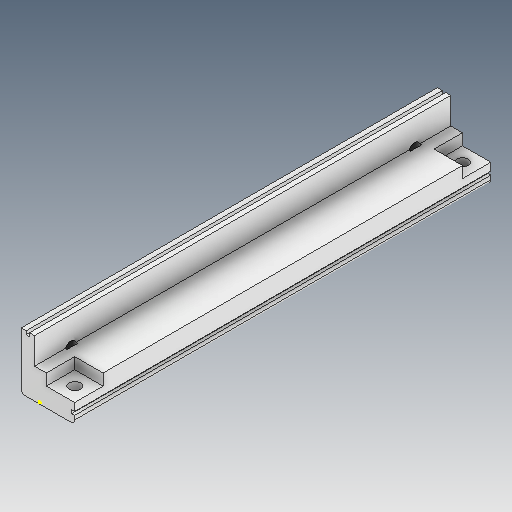
# Autodesk Inventor part: top_edge
Saved by Autodesk Inventor 2027 (Build 310192060, 192F)
## iProperties
Created: 2026-07-26
Part Number: top_edge
Material: ABS Plastic
Document SubType Name: Modeling
Designer: prest
Density: 1.06 g/cm^3
Appearance: Smooth - White
Author: prest
Autodesk Inventor part; units mm, degrees
ref_plane "YZ Plane" through (0, 0, 0) normal (1, 0, 0) x (0, 1, 0)
ref_plane "XZ Plane" through (0, 0, 0) normal (0, 1, 0) x (-1, 0, 0)
ref_plane "XY Plane" through (0, 0, 0) normal (0, 0, 1) x (1, 0, 0)
sketch "Sketch1" plane through (0, 0, 0) normal (0, 1, 0) x (-1, 0, 0)
  line L0 (18.1065, 110) -> (-18.1065, 110)
  line L1 (-18.1065, 110) -> (-18.1065, -110)
  line L2 (-18.1065, -110) -> (18.1065, -110)
  line L3 (18.1065, -110) -> (18.1065, 110)
  point P0 (0, 0)
  point P1 (0, 110)
  point P2 (18.1065, 0)
  dimension "d0" = 220
  dimension "d1" = 36.213
  constraints: 8 end point, 2 midpoint, 2 parallel, 1 horizontal, 1 horizontal alignment, 1 perpendicular, 1 vertical alignment
  measures "d0" distance of L2.end L0.start
  measures "d1" distance of L0.start L0.end
extrude "Extrusion1" add sketch "Sketch1" along normal blind 15
sketch "Sketch2" plane through (0, 15, 0) normal (0, 1, 0) x (1, 0, 0)
  line L0 (-18.1065, 110) -> (-18.1065, -110) projected
  line L1 (18.1065, 110) -> (-18.1065, 110) projected
  line L2 (-18.1065, -110) -> (-3.1065, -110)
  line L3 (-3.1065, -110) -> (-3.1065, 110)
  line L4 (-3.1065, 110) -> (-18.1065, 110)
  line L5 (-18.1065, 110) -> (-18.1065, -110)
  point P0 (0, 0)
  dimension "d4" = 15
  constraints: 8 end point, 2 parallel, 1 horizontal, 1 perpendicular, 1 point on line
  measures "d4" distance of L4.end L3.end
extrude "Extrusion2" add sketch "Sketch2" along normal blind 14
sketch "Sketch3" plane through (0, 15, 0) normal (0, 1, 0) x (1, 0, 0)
  line L0 (-18.1065, -110) -> (18.1065, -110) projected
  line L1 (18.1065, -110) -> (3.1065, -110)
  line L2 (3.1065, -110) -> (3.1065, -95)
  line L3 (3.1065, -95) -> (18.1065, -95)
  line L4 (18.1065, -95) -> (18.1065, -110)
  point P0 (0, 0)
  dimension "d7" = 15
  dimension "d8" = 15
  constraints: 8 end point, 2 parallel, 1 horizontal, 1 perpendicular
  measures "d7" distance of L2.end L3.end
  measures "d8" distance of L1.end L2.end
extrude "Extrusion3" cut sketch "Sketch3" against normal blind 6
mirror "Mirror1" about plane through (0, 0, 0) normal (0, 0, 1) of "Extrusion3"
sketch "Sketch4" plane through (0, 9, 0) normal (0, 1, 0) x (1, 0, 0)
  line L0 (18.1065, -95) -> (18.1065, -110) projected
  line L1 (18.1065, -110) -> (3.1065, -110) projected
  point P0 (0, 0)
  point P1 (10.6065, -102.5)
  point P2 (18.1065, -102.5)
  dimension "d11" = 7.5
  dimension "d12" = 7.5
  constraints: 1 midpoint
  measures "d11" distance of point (18.107, -102.5) point (10.607, -102.5)
  measures "d12" distance from line of L1 point (10.607, -102.5)
hole "Hole1" at (10.6065, 9, 102.5) direction (0, -1, 0) diameter 6 depth 5
mirror "Mirror2" about plane through (0, 0, 0) normal (0, 0, 1) of "Hole1"
sketch "Sketch5" plane through (-18.1065, 0, 110) normal (0, 0, 1) x (1, 0, 0)
  point P0 (18.1065, 0)
move faces "Move2" translate (7.929, 0, 0) faces at (-18.1065, 9.6667, -36.6667)
move faces "Move3" translate (0, -1, 0) faces at (8.6785, 0, 36.6667)
sketch "Sketch6" plane through (18.1065, 9, 95) normal (1, 0, 0) x (0, 0, -1)
  line L0 (205, -10) -> (205, 0) projected
  line L1 (-15, -10) -> (-15, 0) projected
  line L2 (205, -5.9) -> (-15, -5.9)
  line L3 (205, -5) -> (-15, -5)
  line L4 (205, -4.1) -> (-15, -4.1)
  line L5 (205, -4.1) -> (205, -5.9)
  line L6 (205, -10) -> (205, 20) projected
  line L7 (-15, -4.1) -> (-15, -5.9)
  point P0 (95, -9)
  dimension "d29" = 1.8
  constraints: 10 end point, 2 collinear, 2 midpoint, 2 point on line, 2 symmetric about line, 1 perpendicular
  measures "d29" diameter of L2 L3
extrude "Extrusion4" cut sketch "Sketch6" against normal blind 1.6
sketch "Sketch7" plane through (0, 29, 0) normal (0, 1, 0) x (1, 0, 0)
  line L0 (-6.642, 113.6406) -> (-6.642, -120.3961) construction
  line L1 (-3.1065, 110) -> (-10.1775, 110) projected
  line L2 (18.1065, 110) -> (-10.1775, 110) projected
  line L3 (-5.742, 110) -> (-5.742, -110)
  line L4 (-10.1775, -110) -> (-3.1065, -110) projected
  line L5 (-7.542, 110) -> (-7.542, -110)
  line L6 (-5.742, 110) -> (-7.542, 110)
  line L7 (-5.742, -110) -> (-7.542, -110)
  point P0 (0, 0)
  point P1 (-6.642, 110)
  point P2 (-7.542, 110)
  point P3 (-7.542, -110)
  point P4 (-5.742, 110)
  dimension "d35" = 1.8
  constraints: 10 end point, 3 point on line, 2 collinear, 2 symmetric about line, 1 midpoint, 1 parallel, 1 vertical
  measures "d35" diameter of L3 L0
extrude "Extrusion5" cut sketch "Sketch7" against normal blind 1.8
sketch "Sketch16" plane through (-10.1775, 29, -110) normal (-1, 0, 0) x (0, 0, 1)
  line L0 (0, -30) -> (0, 0) projected
  line L1 (220, -30) -> (220, 0) projected
  line L2 (0, 0) -> (220, 0) projected
  point P0 (110, -29)
  point P1 (19.142, -15)
  point P2 (200.858, -15)
  dimension "d75" = 181.716
  dimension "d76" = 220
  dimension "d77" = 19.142
  dimension "d78" = 30
  dimension "d79" = 15
  constraints: 1 horizontal alignment
  measures "d75" distance of point (19.142, -15) point (200.858, -15)
  measures "d76" distance between parallel lines of L0 L1
  measures "d77" distance from line of point (200.858, -15) L1
  measures "d78" distance of L1.start L1.end
  measures "d79" distance from line of L2 point (200.858, -15)
hole "Hole6" at (-10.1775, 14, 90.858) at (-10.1775, 14, -90.858) direction (1, 0, 0) diameter 6 depth 8
fillet "Fillet1" radius 2 1 edges at (-10.1775, -1, 0)
fillet "Fillet2" radius 2 1 edges at (18.1065, -1, 0)
equation "\"d8\" = d7"
equation "\"d11\" = 0.5 * d7"
equation "\"d12\" = 0.5 * d8"
equation "\"d77\" = -0.5 * d75 + 0.5 * d76"
equation "\"d79\" = 0.5 * d78"
body "Solid1"
